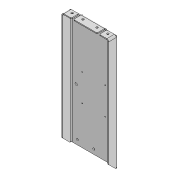
# Autodesk Inventor part: Display_Angle_B
Saved by Autodesk Inventor 2020 (Build 240168000, 168)
## iProperties
Created: 2021-04-28
Part Number: Display_Angle_B
Material: 一般
Document SubType Name: Sheet Metal
Designer: ken113
Density: 1 g/cm^3
Sheet Metal Rule: Default_mm
Appearance: 既定
Author: ken113
Autodesk Inventor part; units mm, degrees
note: some values were not read from the file. Chosen so that the rebuilt part matches the saved one: flange form of "プレート2".
ref_plane "YZ Plane" through (0, 0, 0) normal (1, 0, 0) x (0, 1, 0)
ref_plane "XZ Plane" through (0, 0, 0) normal (0, 1, 0) x (-1, 0, 0)
ref_plane "XY Plane" through (0, 0, 0) normal (0, 0, 1) x (1, 0, 0)
sketch "スケッチ1" plane through (0, 0, 0) normal (0, 0, 1) x (1, 0, 0)
  line L0 (-50, 0) -> (50, 0)
  line L1 (50, 0) -> (50, -242)
  line L2 (50, -242) -> (-50, -242)
  line L3 (-50, -242) -> (-50, 0)
  point P0 (0, 0)
  dimension "d0" = 100
  dimension "d1" = 50
  dimension "d2" = 242
  measures "d0" distance of L1.end L2.end
  measures "d1" distance from line of point (0, 0) L3
  measures "d2" distance of L0.end L1.end
extrude "プレート1" add sketch "スケッチ1" along normal blind 2
sketch "スケッチ2" plane through (48, 0, 0) normal (1, 0, 0) x (0, 1, 0)
  line L0 (-242, 0) -> (0, 0)
  line L1 (0, 0) -> (0, 20)
  line L2 (0, 20) -> (-242, 20)
  line L3 (-242, 20) -> (-242, 0)
  constraints: 6 end point, 1 horizontal, 1 perpendicular, 1 vertical
edge flange "フランジ1" height 20 angle 90 thickness 2 bend radius 2 thickness toward (1, 0, 0) relief tear relief width 2 relief depth 1 corner gap 2 corner form 0 edges at (50, -121, 2) (-50, -121, 2) wall of the first edge with corners at (48, -242, 0) (48, 0, 0) (48, 0, 20) (48, -242, 20)
bend "曲げ1"
corner "コーナー1"
sketch "スケッチ6" plane through (-46, 2, 20) normal (0, 1, 0) x (-1, 0, 0)
  line L0 (0, -16) -> (0, 0)
  line L1 (0, 0) -> (-16, 0)
  line L2 (-16, 0) -> (-16, -16)
  line L3 (-16, -16) -> (0, -16)
  constraints: 6 end point, 1 horizontal, 1 perpendicular, 1 vertical
edge flange "フランジ5" height 20 angle 90 thickness 2 bend radius 2 thickness toward (0, 1, 0) relief tear relief width 2 relief depth 1 corner gap 2 corner form 0 edges at (-48, 0, 12) (48, 0, 12) wall of the first edge with corners at (-46, 2, 4) (-46, 2, 20) (-30, 2, 20) (-30, 2, 4)
bend "曲げ5"
corner "コーナー5"
sketch "スケッチ7" plane through (0, 0, 2) normal (0, 0, 1) x (1, 0, 0)
  line L0 (-25, 0) -> (25, 0)
  line L1 (25, 0) -> (25, 2)
  line L2 (25, 2) -> (-25, 2)
  line L3 (-25, 2) -> (-25, 0)
  line L4 (-30, 2) -> (-30, 4) projected
  line L5 (30, 2) -> (30, 4) projected
  point P0 (0, 0)
  dimension "d55" = 2
  dimension "d56" = 5
  dimension "d57" = 5
  constraints: 8 end point, 2 parallel, 1 horizontal, 1 perpendicular
  measures "d55" distance of L0.end L1.end
  measures "d56" distance between parallel lines of L4 L3
  measures "d57" distance between parallel lines of L5 L1
extrude "押し出し1" add sketch "スケッチ7" against normal up to surface (2 mm away)
sketch "スケッチ8" plane through (-25, 2, 2) normal (0, 1, 0) x (-1, 0, 0)
  line L0 (-50, 0) -> (0, 0)
  line L1 (0, 0) -> (0, 18)
  line L2 (0, 18) -> (-50, 18)
  line L3 (-50, 18) -> (-50, 0)
  constraints: 6 end point, 1 horizontal, 1 perpendicular, 1 vertical
edge flange "フランジ6" height 20 angle 90 thickness 2 bend radius 2 thickness toward (0, 1, 0) relief tear relief width 2 relief depth 1 edges at (0, 2, 2) wall of the first edge with corners at (25, 2, 2) (-25, 2, 2) (-25, 2, 20) (25, 2, 20)
bend "曲げ6"
corner "コーナー6"
sketch "スケッチ9" plane through (0, 0, 2) normal (0, 0, 1) x (1, 0, 0)
  line L0 (25, 4) -> (-25, 4) projected
  point P0 (0, 0)
  point P1 (-37.5, -131)
  point P2 (37.5, -131)
  dimension "d71" = 75
  dimension "d72" = 37.5
  dimension "d73" = 135
  constraints: 1 horizontal alignment
  measures "d71" distance of point (37.5, -131) point (-37.5, -131)
  measures "d72" horizontal distance of point (0, 0) point (-37.5, -131)
  measures "d73" distance from line of point (37.5, -131) L0
hole "穴1" at (-37.5, -131, 2) at (37.5, -131, 2) direction (0, 0, -1) diameter 5.2 depth 2 tip angle 118
chamfer "面取り1" distance 15 angle 45 2 edges at (-49, -242, 20) (49, -242, 20)
fillet "フィレット1" radius 2 6 edges at (-25, 3, 20) (-30, 3, 20) (-30, 3, 4) (25, 3, 20) (30, 3, 4) (30, 3, 20)
sketch "スケッチ10" plane through (-46, 2, 4) normal (0, -1, 0) x (1, 0, 0)
  arc A0 (76, 2) -> (78, 0) centre (78, 2) ccw projected
  line L0 (78, 0) -> (92, 0) projected
  line L1 (92, 0) -> (92, 16) projected
  line L2 (78, 16) -> (92, 16) projected
  arc A1 (78, 16) -> (76, 14) centre (78, 14) ccw projected
  line L3 (76, 14) -> (76, 2) projected
  arc A2 (71, 14) -> (69, 16) centre (69, 14) ccw projected
  line L4 (69, 16) -> (23, 16) projected
  arc A3 (23, 16) -> (21, 14) centre (23, 14) ccw projected
  line L5 (21, 0) -> (21, 14) projected
  line L6 (21, 0) -> (71, 0) projected
  line L7 (71, 0) -> (71, 14) projected
  arc A4 (14, 0) -> (16, 2) centre (14, 2) ccw projected
  line L8 (16, 2) -> (16, 14) projected
  arc A5 (16, 14) -> (14, 16) centre (14, 14) ccw projected
  line L9 (14, 16) -> (0, 16) projected
  line L10 (0, 16) -> (0, 0) projected
  line L11 (14, 0) -> (0, 0) projected
  point P0 (46, -4)
  point P1 (8, 6)
  point P2 (31, 6)
  point P3 (61, 6)
  point P4 (84, 6)
  dimension "d85" = 10
  dimension "d86" = 8
  dimension "d87" = 8
  dimension "d88" = 10
  dimension "d89" = 10
  constraints: 3 horizontal alignment
  measures "d85" distance from line of L9 point (8, 6)
  measures "d86" distance from line of L8 point (8, 6)
  measures "d87" distance from line of point (84, 6) L3
  measures "d88" distance from line of point (31, 6) L5
  measures "d89" distance from line of L7 point (61, 6)
hole "穴2" at (-38, 2, 10) at (-15, 2, 10) at (15, 2, 10) at (38, 2, 10) direction (0, 1, 0) diameter 4.2 depth 2 tip angle 118
sketch "スケッチ11" plane through (0, 0, 2) normal (0, 0, 1) x (1, 0, 0)
  line L0 (24.5, -160) -> (-24.5, -160)
  line L1 (-24.5, -160) -> (-24.5, -102)
  line L2 (-24.5, -102) -> (24.5, -102)
  line L3 (24.5, -102) -> (24.5, -160)
  line L4 (24.5, -160) -> (-24.5, -102) construction
  line L5 (-24.5, -160) -> (24.5, -102) construction
  line L6 (-25, 0) -> (25, 0) projected
  circle A0 centre (-37.5, -131) radius 2.6 projected
  point P0 (0, 0)
  point P1 (0, -131)
  point P2 (0, -131)
  point P3 (0, 0)
  point P4 (0, -131)
  dimension "d97" = 58
  dimension "d98" = 49
  constraints: 12 end point, 5 midpoint, 2 parallel, 1 horizontal, 1 horizontal alignment, 1 perpendicular, 1 vertical alignment
  measures "d97" distance of L0.end L1.end
  measures "d98" distance of L1.end L2.end
hole "穴3" at (-24.5, -160, 2) at (24.5, -160, 2) at (24.5, -102, 2) at (-24.5, -102, 2) direction (0, 0, -1) diameter 2.013 depth 7.6 tip angle 118 thread size "M2.5x0.45" class "6H" standard "ISO Metric profile"
sketch "スケッチ12" plane through (0, 0, 2) normal (0, 0, 1) x (1, 0, 0)
  circle A0 centre (24.5, -102) radius 1.0065 projected
  circle A1 centre (-24.5, -160) radius 1.0065 projected
  circle A2 centre (24.5, -160) radius 1.0065 projected
  circle A3 centre (-24.5, -102) radius 1.0065 projected
  circle A4 centre (-37.5, -131) radius 2.6 projected
  circle A5 centre (37.5, -131) radius 2.6 projected
  line L0 (-46, 0) -> (-25, 0) projected
  line L1 (-46, 0) -> (-46, -242) projected
  line L2 (46, -242) -> (-46, -242) projected
  line L3 (46, -242) -> (46, 0) projected
  line L4 (25, 0) -> (46, 0) projected
  line L5 (-25, 0) -> (25, 0) projected
  point P0 (0, 0)
  point P1 (-35, -232)
  point P2 (35, -232)
  point P3 (0, -232)
  point P4 (0, 0)
  dimension "d106" = 10
  dimension "d107" = 35
  dimension "d108" = 70
  constraints: 2 horizontal alignment, 1 midpoint, 1 vertical alignment
  measures "d106" distance from line of point (-35, -232) L2
  measures "d107" distance of point (0, -232) point (-35, -232)
  measures "d108" distance of point (-35, -232) point (35, -232)
hole "穴4" at (-35, -232, 2) at (35, -232, 2) at (0, -232, 2) direction (0, 0, -1) diameter 4.2 depth 2 tip angle 118
equation "\"d72\" = 0.5 * d71"
equation "\"d79\" = Thickness"
equation "\"d95\" = Thickness"
equation "\"d114\" = Thickness"
equation "\"d3\" = Thickness"
equation "\"d4\" = BendReliefWidth"
equation "\"d5\" = BendReliefDepth"
equation "\"d6\" = MinimumRemnant"
equation "\"d7\" = TransitionRadius"
equation "\"d10\" = BendRadius"
equation "\"d11\" = CornerReliefSize"
equation "\"d12\" = GapSize"
equation "\"d13\" = JacobiRadiusSize"
equation "\"d45\" = BendReliefWidth"
equation "\"d46\" = BendReliefDepth"
equation "\"d47\" = MinimumRemnant"
equation "\"d48\" = TransitionRadius"
equation "\"d51\" = BendRadius"
equation "\"d52\" = CornerReliefSize"
equation "\"d53\" = GapSize"
equation "\"d54\" = JacobiRadiusSize"
equation "\"d60\" = BendReliefWidth"
equation "\"d61\" = BendReliefDepth"
equation "\"d62\" = MinimumRemnant"
equation "\"d63\" = TransitionRadius"
equation "\"d66\" = BendRadius"
equation "\"d68\" = CornerReliefSize"
equation "\"d69\" = GapSize"
equation "\"d70\" = JacobiRadiusSize"
equation "\"d1\" = 0.5 * d0"
equation "\"BendRadius\" = Thickness"
equation "\"BendReliefWidth\" = Thickness"
equation "\"BendReliefDepth\" = 0.5 * Thickness"
equation "\"CornerReliefSize\" = 4 * Thickness"
equation "\"MinimumRemnant\" = 2 * Thickness"
equation "\"TransitionRadius\" = BendRadius"
equation "\"JacobiRadiusSize\" = BendRadius"
equation "\"GapSize\" = Thickness"
equation "\"Thickness\" = 2"
